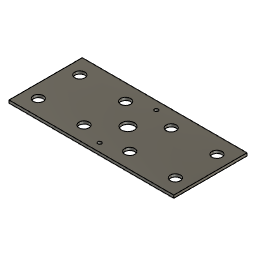
sound-camera (Autodesk Fusion 360 design; units mm, degrees)
Autodesk Fusion 360 part; units mm, degrees
sketch "Sketch1" plane through (0, 0, 0) normal (0, 0, 1) x (1, 0, 0)
  line L0 (-90, 40) -> (90, 40)
  line L1 (90, 40) -> (90, -40)
  line L2 (90, -40) -> (-90, -40)
  line L3 (-90, -40) -> (-90, 40)
  line L4 (-90, 40) -> (90, -40) construction
  line L5 (90, 40) -> (-90, -40) construction
  circle A0 centre (-25, 22.3325) radius 5.5
  circle A1 centre (-75, 22.3727) radius 5.5
  circle A2 centre (-25.3826, -22.6675) radius 5.5
  circle A3 centre (75, 22.1737) radius 5.5
  circle A4 centre (25, 22.2838) radius 5.5
  circle A5 centre (-75.3826, -22.6273) radius 5.5
  circle A6 centre (24.6174, -22.7162) radius 5.5
  circle A7 centre (74.6174, -22.8263) radius 5.5
  circle A8 centre (0, 0) radius 7
  point P0 (-90, 40)
  point P1 (-24.0015, 35.2175)
  dimension "d1" = 80
  dimension "d2" = 180
  dimension "d3" = 11
  dimension "d4" = 11
  dimension "d5" = 11
  dimension "d7" = 11
  dimension "d8" = 11
  dimension "d9" = 11
  dimension "d11" = 11
  dimension "d12" = 11
  dimension "d15" = 50
  dimension "d16" = 50
  dimension "d17" = 50
  dimension "d18" = 50
  dimension "d19" = 50
  dimension "d20" = 50
  dimension "d21" = 45
  dimension "d22" = 45
  dimension "d23" = 45
  dimension "d25" = 45
  dimension "d26" = 14
  constraint horizontal L0
  constraint perpendicular L0 L1
  constraint parallel L0 L2
  constraint parallel L1 L3
  constraint coincident L4 A8.centre
  constraint coincident L5 A8.centre
  constraint coincident A8.centre origin
  measures "d1" distance of L0.end L1.end
  measures "d2" distance of P0 L0.end
  measures "d3" diameter of A0
  measures "d4" diameter of A1
  measures "d5" diameter of A2
  measures "d7" diameter of A3
  measures "d8" diameter of A4
  measures "d9" diameter of A5
  measures "d11" diameter of A6
  measures "d12" diameter of A7
  measures "d15" horizontal distance of A0.centre A1.centre
  measures "d16" horizontal distance of A0.centre A4.centre
  measures "d17" horizontal distance of A4.centre A3.centre
  measures "d18" horizontal distance of A2.centre A5.centre
  measures "d19" horizontal distance of A2.centre A6.centre
  measures "d20" horizontal distance of A6.centre A7.centre
  measures "d21" vertical distance of A0.centre A2.centre
  measures "d22" vertical distance of A4.centre A6.centre
  measures "d23" vertical distance of A3.centre A7.centre
  measures "d25" vertical distance of A1.centre A5.centre
  measures "d26" diameter of A8
extrude "Extrude1" add sketch "Sketch1" along normal blind 7
sketch "Sketch3" plane through (0, 0, 7) normal (0, 0, 1) x (-1, 0, 0)
  circle A0 centre (75.3826, 22.6273) radius 5.5
  circle A1 centre (-74.6174, 22.8263) radius 5.5
  circle A2 centre (0, 0) radius 7
  circle A3 centre (75, -22.3727) radius 5.5
  circle A4 centre (25, -22.3325) radius 5.5
  circle A5 centre (-75, -22.1737) radius 5.5
  circle A6 centre (-24.6174, 22.7162) radius 5.5
  circle A7 centre (-25, -22.2838) radius 5.5
  circle A8 centre (25.3826, 22.6675) radius 5.5
  line L0 (90, 40) -> (-90, 40)
  line L1 (-90, 40) -> (-90, -40)
  line L2 (-90, -40) -> (90, -40)
  line L3 (90, -40) -> (90, 40)
  circle A9 centre (0, -31) radius 2
  line L4 (-20, 0) -> (-2.5, 0)
  circle A10 centre (0, 31) radius 2
  dimension "d29" = 4
  dimension "d30" = 31
  constraint vertical A2.centre A9.centre
  constraint symmetric A9 L4 A10
  measures "d29" diameter of A9
  measures "d30" distance of A2.centre A9.centre
extrude "Extrude2" cut sketch "Sketch3" against normal blind 14 contours A9 | A10
extrude "Extrude3" cut 1 faces at (-43.1381, 6.099, 7) along direction (0, 0, -1) blind 4
equation "d30 = 27 mm + 4 mm"
